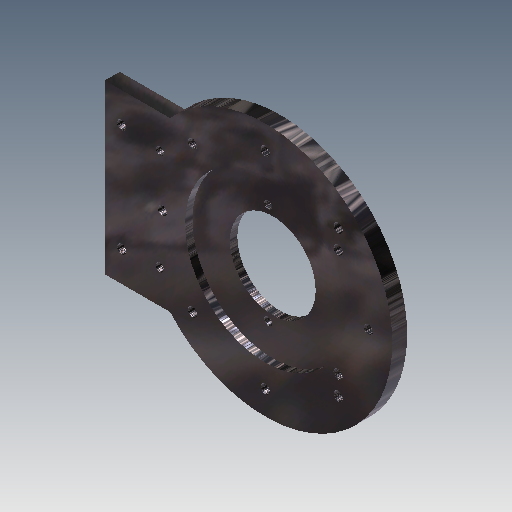
# Autodesk Inventor part: 先端モータマウントC
Saved by Autodesk Inventor 2019.4 (Build 234330000, 330)
## iProperties
Created: 2018-08-10
Part Number: 先端モータマウントC
Material: アルミニウム 6061
Document SubType Name: Modeling
Designer: Owner
Mass: 39.0796 g
Surface Area: 116.368 cm^2
Volume: 14.4739 cm^3
Density: 2.7 g/cm^3
Appearance: アルミニウム - フラット
Author: Owner
Autodesk Inventor part; units mm, degrees
ref_plane "YZ Plane" through (0, 0, 0) normal (1, 0, 0) x (0, 1, 0)
ref_plane "XZ Plane" through (0, 0, 0) normal (0, 1, 0) x (-1, 0, 0)
ref_plane "XY Plane" through (0, 0, 0) normal (0, 0, 1) x (1, 0, 0)
sketch "スケッチ1" plane through (0, 0, 0) normal (0, 0, 1) x (1, 0, 0)
  line L0 (22.7979, -11.619) -> (22.7979, 11.619) construction
  arc A0 (22.7979, 11.619) -> (11.7979, 16) centre (11.7979, 0) ccw construction
  line L1 (11.7979, 16) -> (-18.2021, 16) construction
  arc A1 (-18.2021, 16) -> (-20.2021, 14) centre (-18.2021, 14) ccw construction
  line L2 (-20.2021, 14) -> (-20.2021, -14) construction
  arc A2 (-20.2021, -14) -> (-18.2021, -16) centre (-18.2021, -14) ccw construction
  line L3 (-18.2021, -16) -> (11.7979, -16) construction
  arc A3 (11.7979, -16) -> (22.7979, -11.619) centre (11.7979, 0) ccw construction
  circle A4 centre (-17.4618, -13.5) radius 1.05 construction
  circle A5 centre (-17.4618, 13.5) radius 1.05 construction
  circle A6 centre (9.5382, -13.5) radius 1.05 construction
  circle A7 centre (9.5382, 13.5) radius 1.05 construction
  circle A8 centre (10.7975, 0) radius 2.7 projected
  circle A9 centre (-57.7021, 15) radius 1.6 construction
  circle A10 centre (-27.7021, 15) radius 1.6 construction
  line L4 (-65.2021, 7.5) -> (-65.2021, 22.5) projected
  line L5 (-65.2021, 7.5) -> (-20.2021, 7.5) construction
  line L6 (-20.2021, 22.5) -> (-20.2021, 7.5) construction
  line L7 (-65.2021, 22.5) -> (-20.2021, 22.5) projected
  circle A11 centre (-57.7021, -15) radius 1.6 construction
  circle A12 centre (-27.7021, -15) radius 1.6 construction
  line L8 (-65.2021, -22.5) -> (-65.2021, -7.5) projected
  line L9 (-65.2021, -22.5) -> (-20.2021, -22.5) projected
  line L10 (-20.2021, -7.5) -> (-20.2021, -22.5) construction
  line L11 (-65.2021, -7.5) -> (-20.2021, -7.5) construction
  circle A13 centre (-57.7021, -15) radius 1.6 construction
  circle A14 centre (-57.7021, 15) radius 1.6 construction
  line L12 (-50.2021, -22.5) -> (-65.2021, -22.5) projected
  line L13 (-50.2021, -22.5) -> (-50.2021, 22.5) construction
  line L14 (-65.2021, 22.5) -> (-50.2021, 22.5) projected
  line L15 (-65.2021, -22.5) -> (-65.2021, 22.5) projected
  circle A15 centre (10.7975, 0) radius 27.5 construction
  line L16 (-65.2021, 22.5) -> (-14.7118, 22.5)
  line L17 (-65.2021, 22.5) -> (-65.2021, -22.5)
  line L18 (-65.2021, -22.5) -> (-14.7118, -22.5)
  arc A16 (-14.7118, -22.5) -> (-14.7118, 22.5) centre (10.7975, 0) ccw
  circle A17 centre (10.7975, 0) radius 11.5
  circle A18 centre (9.5382, 13.5) radius 1.1
  circle A19 centre (9.5382, -13.5) radius 1.1
  circle A20 centre (-17.4618, 13.5) radius 1.1
  circle A21 centre (-17.4618, -13.5) radius 1.1
  circle A22 centre (-27.7021, 15) radius 1.25
  circle A23 centre (-57.7021, 15) radius 1.25
  circle A24 centre (-57.7021, -15) radius 1.25
  circle A25 centre (-27.7021, -15) radius 1.25
  point P0 (0, 0)
  dimension "d0" = 55
  dimension "d1" = 23
  dimension "d2" = 2.2
  dimension "d3" = 2.2
  dimension "d4" = 2.2
  dimension "d5" = 2.2
  dimension "d6" = 2.5
  dimension "d7" = 2.5
  dimension "d8" = 2.5
  dimension "d9" = 2.5
  constraints: 11 centre point, 11 coincident, 6 end point, 2 perpendicular, 2 point on circle, 1 point on line
  measures "d0" diameter of A15
  measures "d1" diameter of A17
  measures "d2" diameter of A18
  measures "d3" diameter of A19
  measures "d4" diameter of A20
  measures "d5" diameter of A21
  measures "d6" diameter of A22
  measures "d7" diameter of A23
  measures "d8" diameter of A24
  measures "d9" diameter of A25
extrude "押し出し1" add sketch "スケッチ1" along normal blind 4 contours L4 L7 L16 A16 L18 L9 L8 L15
sketch "スケッチ2" plane through (0, 0, 4) normal (0, 0, 1) x (1, 0, 0)
  circle A0 centre (10.7975, 0) radius 11.5 projected
  circle A1 centre (-27.7021, -15) radius 1.25 projected
  circle A2 centre (-57.7021, -15) radius 1.25 projected
  circle A3 centre (-57.7021, 15) radius 1.25 projected
  circle A4 centre (-27.7021, 15) radius 1.25 projected
  circle A5 centre (-17.4618, -13.5) radius 1.1 projected
  circle A6 centre (-17.4618, 13.5) radius 1.1 projected
  circle A7 centre (9.5382, -13.5) radius 1.1 projected
  circle A8 centre (9.5382, 13.5) radius 1.1 projected
  line L0 (-65.2021, 22.5) -> (-65.2021, -22.5) projected
  line L1 (-65.2021, -22.5) -> (-14.7118, -22.5) projected
  arc A9 (-14.7118, -22.5) -> (-14.7118, 22.5) centre (10.7975, 0) ccw projected
  line L2 (-14.7118, 22.5) -> (-65.2021, 22.5) projected
  circle A10 centre (10.7975, 0) radius 21.5
  point P0 (0, 0)
  dimension "d12" = 43
  constraints: 1 centre point, 1 coincident
  measures "d12" diameter of A10
extrude "押し出し4" cut sketch "スケッチ2" against normal blind 2 contours A10
sketch "スケッチ4" plane through (0, 0, 4) normal (0, 0, 1) x (1, 0, 0)
  circle A0 centre (10.7975, 0) radius 21.5 projected
  circle A1 centre (-27.7021, -15) radius 1.25 projected
  circle A2 centre (-57.7021, -15) radius 1.25 projected
  circle A3 centre (-57.7021, 15) radius 1.25 projected
  circle A4 centre (-27.7021, 15) radius 1.25 projected
  circle A5 centre (-17.4618, -13.5) radius 1.1 projected
  circle A6 centre (-17.4618, 13.5) radius 1.1 projected
  line L0 (-65.2021, 22.5) -> (-65.2021, -22.5) projected
  line L1 (-65.2021, -22.5) -> (-14.7118, -22.5) projected
  arc A7 (-14.7118, -22.5) -> (-14.7118, 22.5) centre (10.7975, 0) ccw projected
  line L2 (-14.7118, 22.5) -> (-65.2021, 22.5) projected
  circle A8 centre (10.7975, 0) radius 27.6
  circle A9 centre (38.3975, 0) radius 1.25
  circle A10 centre (30.3137, 19.5161) radius 1.25
  circle A11 centre (10.7975, 27.6) radius 1.25
  circle A12 centre (-8.7186, 19.5161) radius 1.25
  circle A13 centre (-16.8025, 0) radius 1.25
  circle A14 centre (-8.7186, -19.5161) radius 1.25
  circle A15 centre (10.7975, -27.6) radius 1.25
  circle A16 centre (30.3137, -19.5161) radius 1.25
  point P0 (0, 0)
  dimension "d25" = 55.2
  dimension "d26" = 2.5
  dimension "d29" = 360
  constraints: 8 centre point, 1 coincident, 1 horizontal alignment, 19 other
  measures "d26" diameter of A9
extrude "押し出し5" cut sketch "スケッチ4" against normal through all contours A8 A9 | A8 A9 | A10 A8 | A8 A10 | A16 A8 | A8 A16 | A11 A8 | A8 A11 | A15 A8 | A8 A15 | A12 A8 | A8 A12 | A14 A8 | A8 A14 | A13 A8 | A8 A13
move faces "移動1" translate (33, 0, 0) faces at (-65.2021, 7.5, 1.3333)
sketch "スケッチ8" plane through (0, 0, 0) normal (0, 0, -1) x (-1, 0, 0)
  circle A0 centre (27.7021, -15) radius 1.25 projected
  circle A1 centre (27.7021, 15) radius 1.25 projected
  point P0 (0, 0)
extrude "押し出し7" add sketch "スケッチ8" against normal blind 4
sketch "スケッチ7" plane through (0, 0, 0) normal (0, 0, -1) x (-1, 0, 0)
  circle A0 centre (-30.2979, -14.4) radius 1.6 projected
  circle A1 centre (-30.2979, 14.4) radius 1.6 projected
  circle A2 centre (27.7021, -14.4) radius 1.6 projected
  circle A3 centre (27.7021, 14.4) radius 1.6 projected
  circle A4 centre (-30.2979, -14.4) radius 1.25
  circle A5 centre (-30.2979, 14.4) radius 1.25
  circle A6 centre (27.7021, -14.4) radius 1.25
  circle A7 centre (27.7021, 14.4) radius 1.25
  point P0 (0, 0)
  dimension "d45" = 2.5
  dimension "d46" = 2.5
  dimension "d47" = 2.5
  dimension "d48" = 2.5
  constraints: 4 centre point, 4 coincident
  measures "d45" diameter of A4
  measures "d46" diameter of A5
  measures "d47" diameter of A6
  measures "d48" diameter of A7
extrude "押し出し8" cut sketch "スケッチ7" against normal through all contours A4 | A5 | A6 | A7
